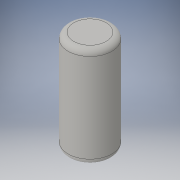
# Autodesk Inventor part: dowel
Saved by Autodesk Inventor 2016 (Build 200138000, 138)
## iProperties
Created: 2019-02-06
Part Number: dowel
Material: Generic
Document SubType Name: Modeling
Designer: Matthew Reese
Density: 1 g/cm^3
Appearance: Default
Author: Matthew Reese
Autodesk Inventor part; units mm, degrees
ref_plane "YZ Plane" through (0, 0, 0) normal (1, 0, 0) x (0, 1, 0)
ref_plane "XZ Plane" through (0, 0, 0) normal (0, 1, 0) x (-1, 0, 0)
ref_plane "XY Plane" through (0, 0, 0) normal (0, 0, 1) x (1, 0, 0)
sketch "Sketch1" plane through (0, 0, 0) normal (0, 0, 1) x (1, 0, 0)
  line L0 (-0.381, -9.136) -> (-0.381, 8.4693)
  line L1 (-6.477, 0) -> (5.715, 0)
  line L2 (-6.477, 0) -> (-6.477, 27.94)
  line L3 (-6.477, 27.94) -> (5.715, 27.94)
  line L4 (5.715, 27.94) -> (5.715, 0)
  point P0 (0, 0)
  dimension "dw" = 12.192
  dimension "d1" = 6.096
  dimension "d2" = 27.94
  constraints: 10 end point, 2 perpendicular, 2 vertical, 1 horizontal
  measures "dw" distance of L1.start L1.end
  measures "d1" distance from line of L1.start L0
  measures "d2" distance of L1.start L2.end
extrude "Extrusion1" add sketch "Sketch1" along normal blind 12.192
fillet "Fillet1" radius 6.096 4 edges at (5.715, 13.97, 12.192) (5.715, 13.97, 0) (-6.477, 13.97, 0) (-6.477, 13.97, 12.192)
fillet "Fillet2" radius 1.5875 3 edges at (5.715, 27.94, 6.096) (3.9297, 27.94, 10.4067) (-0.381, 27.94, 12.192)
fillet "Fillet3" radius 1.5875 3 edges at (-0.381, 0, 12.192) (3.9297, 0, 10.4067) (5.715, 0, 6.096)
equation "\"d1\" = 0.5 * dw"
equation "\"d3\" = dw"
equation "\"d5\" = 0.5 * dw"
body "Solid1"
